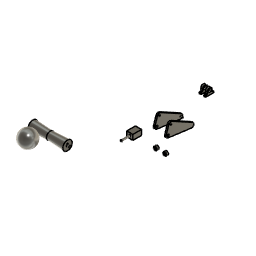
Assembly 1.0 v8 (Autodesk Fusion 360 archive; units mm, degrees)
design "Pinza 4.2"
Autodesk Fusion 360 part; units mm, degrees
note: some values were not read from the file. Chosen so that the rebuilt part matches the saved one: which bodies a step acts on.
box "BoxPrimitive1" add length 18.5 width 13 height 11 placed x (0, 1, 0) y (-1, 0, 0) z (0, 0, 1) at (13, 0, 0) makes body 1
cylinder "CylinderPrimitive1" add diameter 4 height 18.5 placed x (1, 0, 0) y (0, 1, 0) z (0, 0, 1) at (6, -42, 0) separate body makes body 2
copy_body "Body->Comp1" bodies 1 removing the originals makes body 3 in component "Solenoide/Cuerpo"
copy_body "Body->Comp2" bodies 2 removing the originals makes body 4 in component "Solenoide/Vastago"
sketch "Sketch4" plane through (0, 0, 0) normal (1, 0, 0) x (0, 1, 0)
  circle A0 centre (0, 40) radius 2.5
  line L0 (-1, 42.2913) -> (-1, 44)
  line L1 (-1, 44) -> (1, 44)
  line L2 (1, 44) -> (1, 42.2913)
  dimension "d17" = 5
  dimension "d18" = 40
  dimension "d108" = 2
  dimension "d109" = 1
  dimension "d110" = 4
  constraint vertical origin A0.centre
  constraint coincident A0 L0.start
  constraint vertical L0
  constraint perpendicular L0 L1
  constraint coincident A0 L2.end
  constraint perpendicular L1 L2
  measures "d17" diameter of A0
  measures "d18" distance of origin A0.centre
  measures "d108" distance of L0.end L1.end
  measures "d109" horizontal distance of A0.centre L0.end
  measures "d110" distance of A0.centre L1
extrude "Extrude1" add sketch "Sketch4" along normal mid plane 84 separate body contours A0 makes body 5
extrude "Extrude8" add sketch "Sketch4" along normal mid plane 74 contours A0 L0 L1 L2 bodies 5
sketch "Sketch5" plane through (0, 0, 0) normal (0, 1, 0) x (1, 0, 0)
  line L0 (-42, -37.5) -> (-42, -42.5)
  line L1 (42, -42.5) -> (42, -37.5)
  line L2 (-63.1551, -40) -> (60.8449, -40) construction
  line L3 (-37, -40) -> (-37, -50)
  line L4 (-37, -50) -> (0, -48)
  line L5 (0, -48) -> (37, -50)
  line L6 (37, -50) -> (37, -40)
  line L7 (-37, -40) -> (37, -40)
  line L8 (-37, -42.2913) -> (-37, -42.5)
  line L9 (-37, -42.2913) -> (37, -42.2913)
  line L10 (37, -42.5) -> (37, -42.2913)
  line L11 (37, -42.2913) -> (-37, -42.2913)
  dimension "d21" = 2.5
  dimension "d22" = 10
  dimension "d23" = 8
  dimension "d24" = 74
  dimension "d25" = 37
  constraint horizontal L2
  constraint coincident L2 L3.start
  constraint perpendicular L2 L3
  constraint coincident L2 L6.end
  constraint perpendicular L2 L6
  constraint horizontal L3.end L5.end
  constraint vertical origin L4.end
  measures "d21" distance of L0.end L2
  measures "d22" distance of L5.end L6.end
  measures "d23" distance of L4.end L7
  measures "d24" distance of L3.end L5.end
  measures "d25" horizontal distance of origin L3.end
revolve "Revolve1" add sketch "Sketch5" angle 360 about axis through (-63.1551, 0, 40) along (1, 0, 0) separate body makes body 6
combine "Combine1" operation cut target body 6 tool bodies 5 keep tools
split "Split1" by plane through (0, 0, 0) normal (1, 0, 0) bodies 6 makes body 7 at (32.8889, 9.7504, 39.2693)
copy_body "Body->Comp3" bodies 5 removing the originals makes body 8 in component "Rodillo/Eje"
copy_body "Body->Comp4" bodies 6 removing the originals makes body 9 in component "Rodillo/Cono/1"
copy_body "Body->Comp5" bodies 7 removing the originals makes body 10 in component "Rodillo/Cono/2"
sphere "SpherePrimitive1" add diameter 35 placed x (1, 0, 0) y (0, 1, 0) z (0, 0, 1) at (-90, -50, 0) separate body makes body 11
copy_body "Body->Comp6" bodies 11 removing the originals makes body 12 in component "Bola"
sketch "Sketch7" plane through (0, 0, 0) normal (1, 0, 0) x (0, 1, 0)
  line L0 (124.144, 24.0474) -> (73.924, 30.6966)
  line L1 (69.8278, 37.2072) -> (75.4102, 54.2804)
  line L2 (82.5614, 57.1135) -> (127.0089, 32.8094)
  line L3 (128.8918, 28.0567) -> (128.471, 26.7697)
  circle A0 centre (73.9854, 35.2549) radius 2.5
  circle A1 centre (124.8794, 28.6563) radius 1.5
  arc A2 (82.5614, 57.1135) -> (75.4102, 54.2804) centre (80.1626, 52.7265) ccw
  arc A3 (69.8278, 37.2072) -> (73.924, 30.6966) centre (74.5802, 35.6533) ccw
  arc A4 (128.8918, 28.0567) -> (127.0089, 32.8094) centre (125.0898, 29.2998) ccw
  arc A5 (124.144, 24.0474) -> (128.471, 26.7697) centre (124.669, 28.0128) ccw
  line L4 (120.6238, 15.6408) -> (125.2985, 29.9379) construction
  circle A6 centre (80.1626, 52.7265) radius 1.5
  point P0 (127.4383, 23.6113)
  point P1 (67.9573, 31.4866)
  point P2 (77.2807, 60.001)
  point P3 (129.9245, 31.2151)
  dimension "d44" = 5
  dimension "d47" = 30
  dimension "d50" = 8
  dimension "d51" = 60
  dimension "d53" = 60
  dimension "d54" = 3
  dimension "d55" = 5
  dimension "d56" = 5
  dimension "d57" = 4
  dimension "d58" = 4
  dimension "d59" = 0.677
  dimension "d60" = 1.354
  dimension "d121" = 3
  constraint parallel L1 L3
  constraint coincident P2 L1
  constraint coincident P2 L2
  constraint tangent L1 A2
  constraint tangent L2 A2
  constraint coincident P1 L0
  constraint coincident P1 L1
  constraint tangent L0 A3
  constraint tangent L1 A3
  constraint coincident P3 L2
  constraint coincident P3 L3
  constraint tangent L2 A4
  constraint tangent L3 A4
  constraint coincident P0 L0
  constraint coincident P0 L3
  constraint tangent L0 A5
  constraint tangent L3 A5
  constraint coincident A5.centre L4
  constraint coincident A4.centre L4
  constraint coincident A1.centre L4
  constraint concentric A2 A6
  measures "d44" diameter of A0
  measures "d47" distance of P1 P2
  measures "d50" distance of P0 P3
  measures "d51" distance of P2 P3
  measures "d53" distance of P0 P1
  measures "d54" diameter of A1
  measures "d55" radius of A2
  measures "d56" radius of A3
  measures "d57" radius of A4
  measures "d58" radius of A5
  measures "d59" distance of A1.centre A4.centre
  measures "d60" distance of A4.centre A5.centre
  measures "d121" diameter of A6
extrude "Extrude3" add sketch "Sketch7" along normal blind 3 separate body contours L0 L1 L2 L3 A2 A3 A4 A5 | A1 makes body 13
extrude "Extrude7" add sketch "Sketch7" against normal blind 4 contours A1 bodies 13
mirror "Mirror1" about plane through (0, 0, 0) normal (1, 0, 0) of bodies 13 makes body 14
copy_body "Body->Comp15" bodies 14 removing the originals makes body 15 in component "Component''''"
copy_body "Body->Comp16" bodies 13 removing the originals makes body 16 in component "Component'''''"
sketch "Sketch8" plane through (0, 0, 0) normal (1, 0, 0) x (0, 1, 0)
  line L0 (154, 3.0033) -> (154, 5.0033)
  line L1 (155, 6.0033) -> (157, 6.0033)
  line L2 (158, 7.0033) -> (158, 11.5275)
  line L3 (168, 11.5275) -> (168, 7.0033)
  line L4 (169, 6.0033) -> (171, 6.0033)
  line L5 (172, 5.0033) -> (172, 3.0033)
  line L6 (172, 3.0033) -> (154, 3.0033)
  circle A0 centre (163, 11.5275) radius 4
  arc A1 (162.8121, 16.524) -> (158, 11.5275) centre (163, 11.5275) ccw
  arc A2 (168, 11.5275) -> (162.8121, 16.524) centre (163, 11.5275) ccw
  arc A3 (157, 6.0033) -> (158, 7.0033) centre (157, 7.0033) ccw
  arc A4 (168, 7.0033) -> (169, 6.0033) centre (169, 7.0033) ccw
  arc A5 (155, 6.0033) -> (154, 5.0033) centre (155, 5.0033) ccw
  arc A6 (172, 5.0033) -> (171, 6.0033) centre (171, 5.0033) ccw
  point P0 (154, 6.0033)
  point P1 (158, 14.0012)
  point P2 (168, 14.0033)
  point P3 (168, 6.0033)
  point P4 (172, 6.0033)
  dimension "d67" = 18
  dimension "d68" = 10
  dimension "d69" = 4
  dimension "d70" = 8
  dimension "d71" = 3
  dimension "d72" = 8
  dimension "d73" = 5
  dimension "d74" = 5
  dimension "d75" = 1
  dimension "d76" = 1
  dimension "d77" = 1
  dimension "d78" = 1
  constraint vertical L0
  constraint perpendicular L0 L1
  constraint perpendicular L1 L2
  constraint perpendicular L3 L4
  constraint perpendicular L4 L5
  constraint perpendicular L0 L6
  constraint coincident P1 L2
  constraint tangent L2 A1
  constraint coincident P2 L3
  constraint tangent L3 A2
  constraint coincident A1.start A2.end
  constraint coincident A0.centre A1.centre
  constraint tangent L1 A3
  constraint tangent L2 A3
  constraint coincident P3 L3
  constraint coincident P3 L4
  constraint tangent L3 A4
  constraint tangent L4 A4
  constraint coincident P0 L0
  constraint coincident P0 L1
  constraint tangent L0 A5
  constraint tangent L1 A5
  constraint coincident P4 L4
  constraint coincident P4 L5
  constraint tangent L4 A6
  constraint tangent L5 A6
  constraint horizontal L4
  constraint horizontal P3 L1.end
  measures "d67" distance of L0.start L5.end
  measures "d68" distance of P1 P2
  measures "d69" horizontal distance of P0 P1
  measures "d70" distance of P2 P3
  measures "d71" distance of P4 L5.end
  measures "d72" diameter of A0
  measures "d73" radius of A1
  measures "d74" radius of A2
  measures "d75" radius of A3
  measures "d76" radius of A4
  measures "d77" radius of A5
  measures "d78" radius of A6
extrude "Extrude4" add sketch "Sketch8" along normal blind 4 separate body makes body 17
pattern_linear "R-Pattern2" count 2 spacing 10 along (1, 0, 0) of bodies 17 makes body 18
copy_body "Body->Comp9" bodies 17 removing the originals makes body 19 in component "Union/1"
copy_body "Body->Comp10" bodies 18 removing the originals makes body 20 in component "Union/2"
sketch "Sketch9" plane through (0, 0, 0) normal (0, 1, 0) x (1, 0, 0)
  circle A0 centre (81.0005, -9.1416) radius 4
  circle A1 centre (81.0005, -9.1416) radius 1.5
  circle A2 centre (81.0005, -9.1416) radius 2.5
  dimension "d85" = 8
  dimension "d86" = 3
  dimension "d87" = 5
  constraint concentric A0 A1
  constraint concentric A0 A2
  measures "d85" diameter of A0
  measures "d86" diameter of A1
  measures "d87" diameter of A2
extrude "Extrude5" add sketch "Sketch9" along normal blind 4 separate body contours A0 makes body 21
extrude "Extrude6" add sketch "Sketch9" along normal blind 4 separate body contours A2 makes body 22
pattern_linear "R-Pattern3" count 2 spacing 20 along (-1, 0, 0) of bodies 21 22 makes body 23 at (64.9955, 2.6667, 9.341) makes body 24 at (60.3836, 2.6667, 7.7743)
copy_body "Body->Comp11" bodies 21 removing the originals makes body 25 in component "Component"
copy_body "Body->Comp12" bodies 22 removing the originals makes body 26 in component "Component'"
copy_body "Body->Comp13" bodies 23 removing the originals makes body 27 in component "Component''"
copy_body "Body->Comp14" bodies 24 removing the originals makes body 28 in component "Component'''"
component "Solenoide/Cuerpo" placed x (1, 0, 0) y (0, 1, 0) z (0, 0, 1) at (0, 0, 0)
component "Solenoide/Vastago" placed x (1, 0, 0) y (0, 0, -1) z (0, 1, 0) at (0.5, -18.5, -36.5)
component "Rodillo/Eje" placed x (1, 0, 0) y (0, 1, 0) z (0, 0, 1) at (-76.5233, -86.7289, -32.1678)
component "Rodillo/Cono/1" placed x (1, 0, 0) y (0, 1, 0) z (0, 0, 1) at (-76.5233, -86.7289, -32.1678)
component "Rodillo/Cono/2" placed x (1, 0, 0) y (0, 1, 0) z (0, 0, 1) at (-76.5233, -86.7289, -32.1678)
component "Bola" placed x (1, 0, 0) y (0, 1, 0) z (0, 0, 1) at (-5.191, -65.6968, 7.8025)
component "Component''''" placed x (1, 0, 0) y (0, 1, 0) z (0, 0, 1) at (10.4045, -20.4099, -38.1159)
component "Component'''''" placed x (1, 0, 0) y (0, 1, 0) z (0, 0, 1) at (20.964, -9.8513, -52.7134)
component "Union/1" placed x (1, 0, 0) y (0, 1, 0) z (0, 0, 1) at (0, 0, 0)
component "Union/2" placed x (1, 0, 0) y (0, 1, 0) z (0, 0, 1) at (0, 0, 0)
component "Component" placed x (1, 0, 0) y (0, 1, 0) z (0, 0, 1) at (0, 0, 0)
component "Component'" placed x (1, 0, 0) y (0, 1, 0) z (0, 0, 1) at (0, 0, 0)
component "Component''" placed x (1, 0, 0) y (0, 1, 0) z (0, 0, 1) at (0, 0, 0)
component "Component'''" placed x (1, 0, 0) y (0, 1, 0) z (0, 0, 1) at (0, 0, 0)
equation "d3 = ( 37 / 2 ) * 1 mm"
equation "d9 = ( 37 / 2 ) * 1 mm"
equation "d19 = 35 mm + 7 mm"
equation "d24 = ( 37 * 2 ) * 1 mm"
equation "d59 = d60 / 2"
equation "d77 = d75"
equation "d109 = d108 / 2"
